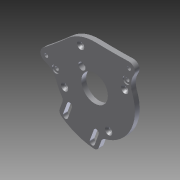
# Autodesk Inventor part: motor plate
Saved by Autodesk Inventor 2012 (Build 160160000, 160)
## iProperties
Created: 2012-02-08
Part Number: motor plate
Material: Default
Document SubType Name: Modeling
Designer: Antonella Wilby
Density: 1 g/cm^3
Author: Antonella Wilby
Autodesk Inventor part; units mm, degrees
ref_plane "YZ Plane" through (0, 0, 0) normal (1, 0, 0) x (0, 1, 0)
ref_plane "XZ Plane" through (0, 0, 0) normal (0, 1, 0) x (-1, 0, 0)
ref_plane "XY Plane" through (0, 0, 0) normal (0, 0, 1) x (1, 0, 0)
sketch "Sketch1" plane through (0, 0, 0) normal (0, 0, 1) x (1, 0, 0)
  line L0 (-661.6722, 0) -> (196.8414, 0) projected
  line L1 (0, -250.3433) -> (0, 987.2762) projected
  line L2 (0, 0) -> (-137.5064, 137.5064) construction
  circle A0 centre (0, 0) radius 17.78
  line L3 (0, 0) -> (46.0238, 46.0238) construction
  line L4 (-64.8398, 5.6727) -> (0, 0) construction
  circle A1 centre (-64.8398, 5.6727) radius 6.35 construction
  circle A2 centre (46.0238, 46.0238) radius 6.35 construction
  arc A3 (52.7316, 41.7801) -> (45.7909, 53.9579) centre (46.0238, 46.0238) ccw
  arc A4 (-69.7613, 11.9003) -> (-67.2505, -1.8898) centre (-64.8398, 5.6727) ccw
  line L5 (0, 0) -> (3.2586, 111.9917) construction
  line L6 (0, 0) -> (-89.6909, 100.7848) construction
  arc A5 (-69.7613, 11.9003) -> (-35.8824, 40.3207) centre (-539.0274, 605.7002) ccw
  arc A6 (1.5698, 53.9522) -> (45.7909, 53.9579) centre (23.5824, 810.4734) ccw
  arc A7 (-50.976, -17.7412) -> (-67.2505, -1.8898) centre (-74.9647, -26.0901) ccw
  arc A8 (52.7316, 41.7801) -> (50.4537, 19.1761) centre (74.1966, 28.2002) ccw
  arc A9 (1.5698, 53.9522) -> (-35.8824, 40.3207) centre (0, 0) ccw
  line L7 (-43.1182, -37.2395) -> (-46.8396, -47.4638)
  line L8 (9.0934, -56.243) -> (5.3721, -66.4673)
  arc A10 (-44.5419, -54.8181) -> (-1.1153, -70.6241) centre (6.0603, 16.6506) ccw
  arc A11 (-50.976, -17.7412) -> (-43.9184, -31.3763) centre (0, 0) ccw
  arc A12 (13.4752, -52.2659) -> (50.4537, 19.1761) centre (0, 0) ccw
  line L9 (-23.8901, -65.6375) -> (0, 0) construction
  arc A13 (-43.1182, -37.2395) -> (-43.9184, -31.3763) centre (-49.0853, -35.0676) ccw
  arc A14 (13.4752, -52.2659) -> (9.0934, -56.243) centre (15.0605, -58.4148) ccw
  arc A15 (-1.1153, -70.6241) -> (5.3721, -66.4673) centre (-0.595, -64.2955) ccw
  arc A16 (-46.8396, -47.4638) -> (-44.5419, -54.8181) centre (-40.8726, -49.6356) ccw
  circle A17 centre (-17.0625, 17.0625) radius 4.7625
  circle A18 centre (0, 0) radius 16.51 construction
  point P0 (-41.9333, -33.9838)
  point P1 (-48.4488, -51.885)
  point P2 (3.7629, -70.8885)
  point P3 (10.2784, -52.9873)
  dimension "d1" = 45
  dimension "d2" = 35.56
  dimension "d33" = 45
  dimension "d34" = 65.0875
  dimension "d39" = 65.0875
  dimension "d40" = 12.7
  dimension "d41" = 130
  dimension "d42" = 1.5875
  dimension "d43" = 1.5875
  dimension "d44" = 43.333
  dimension "d46" = 86.667
  dimension "d47" = 25.4
  dimension "d48" = 53.975
  dimension "d70" = 53.975
  dimension "d71" = 53.975
  dimension "d72" = 20
  dimension "d74" = 19.05
  dimension "d75" = 19.05
  dimension "d76" = 69.85
  dimension "d77" = 27.7812
  dimension "d78" = 6.35
  dimension "d89" = 24.13
  dimension "d90" = 9.525
  dimension "d91" = 33.02
  constraints: 35 point on circle, 19 centre point, 16 end point, 15 tangent, 7 point on line, 6 equal radius, 5 coincident, 2 parallel
  measures "d1" angle of L1 L2
  measures "d2" diameter of A0
  measures "d33" angle of L0 L3
  measures "d34" distance of L3.start L3.end
  measures "d39" distance of L4.start L3.start
  measures "d40" diameter of A1
  measures "d41" angle of L3 L4
  measures "d42" radial gap between concentric circles of A4 A1
  measures "d43" radial gap between concentric circles of A3 A2
  measures "d44" angle of L5 L3
  measures "d46" angle of L6 L3
  measures "d47" radius of A7
  measures "d48" radius of A9
  measures "d70" radius of A11
  measures "d71" radius of A12
  measures "d72" angle of L1 L8
  measures "d74" distance of point (-41.933, -33.984) point (-48.449, -51.885)
  measures "d75" distance of point (10.278, -52.987) point (3.763, -70.888)
  measures "d76" distance of L9.start L3.start
  measures "d77" distance between parallel lines of L9 L8
  measures "d78" radius of A13
  measures "d89" distance of point (0, 0) A17.centre
  measures "d90" diameter of A17
  measures "d91" diameter of A18
extrude "Base" add sketch "Sketch1" along normal mid plane 6.35 contours A4 A5 A9 L1 A0 L0 | L0 A0 L1 A15 A10 A16 L7 A13 A11 A7 A4 | L1 A9 A6 A3 A8 A12 L0 A0 | A0 L0 A12 A14 L8 A15 L1
sketch "Sketch3" plane through (0, 0, 3.175) normal (0, 0, 1) x (1, 0, 0)
  line L0 (0, 0) -> (-18.7854, 40.2854) construction
  line L1 (-98.1278, 0) -> (79.3255, 0) projected
  line L2 (0, -95.5696) -> (0, 78.8991) projected
  point P0 (-40.2854, -18.7854)
  point P1 (18.7854, -40.2854)
  point P2 (40.2854, 18.7854)
  dimension "d20" = 44.45
  dimension "d23" = 360
  dimension "d57" = 25
  constraints: 2 end point, 1 coincident, 5 other
  measures "d20" distance of L0.start L0.end
  measures "d57" angle of L2 L0
hole "Motor Mount Holes" at (-18.7854, 40.2854, 3.175) at (-40.2854, -18.7854, 3.175) at (18.7854, -40.2854, 3.175) at (40.2854, 18.7854, 3.175) direction (0, 0, -1) diameter 5.1054 end through all countersink diameter 9.779 countersink angle 82 clearance for "Flat Head Machine Screw (82)" size "#10" standard "Ansi Unified Screw Threads"
sketch "Sketch4" plane through (0, 0, -3.175) normal (0, 0, -1) x (-1, 0, 0)
  arc A0 (67.2505, -1.8898) -> (69.7613, 11.9003) centre (64.8398, 5.6727) ccw projected
  arc A1 (-45.7909, 53.9579) -> (-52.7316, 41.7801) centre (-46.0238, 46.0238) ccw projected
  constraints: 2 coincident
hole "Standoff holes to back plate" at (46.0238, 46.0238, -3.175) at (-64.8398, 5.6727, -3.175) direction (0, 0, 1) diameter 5.1054 end through all counterbore diameter 9.779 counterbore depth 1.5875 clearance for "Flat Head Machine Screw (82)" size "#10" standard "Ansi Unified Screw Threads"
sketch "Sketch5" plane through (0, 0, 3.175) normal (0, 0, 1) x (1, 0, 0)
  circle A0 centre (-64.8398, 5.6727) radius 2.5527 projected
  circle A1 centre (46.0238, 46.0238) radius 2.5527 projected
  arc A2 (-50.976, -17.7412) -> (-67.2505, -1.8898) centre (-74.9647, -26.0901) ccw projected
  arc A3 (52.7316, 41.7801) -> (50.4537, 19.1761) centre (74.1966, 28.2002) ccw projected
  circle A4 centre (-52.2111, -3.9465) radius 6.35 construction
  circle A5 centre (42.5328, 30.5374) radius 6.35 construction
  dimension "d58" = 15.875
  dimension "d59" = 15.875
  dimension "d60" = 12.7
  dimension "d62" = 12.7
  constraints: 2 centre point, 2 coincident, 2 tangent
  measures "d58" distance of A0.centre point (-52.211, -3.947)
  measures "d59" distance of point (42.533, 30.537) A1.centre
  measures "d60" diameter of A4
  measures "d62" diameter of A5
hole "Standoff holes to front plate" at (-52.2111, -3.9465, 3.175) at (42.5328, 30.5374, 3.175) direction (0, 0, -1) diameter 5.1054 end through all counterbore diameter 9.779 counterbore depth 1.5875 clearance for "Flat Head Machine Screw (82)" size "#10" standard "Ansi Unified Screw Threads"
sketch "Sketch6" plane through (0, 0, 3.175) normal (0, 0, 1) x (1, 0, 0)
  arc A0 (-44.5419, -54.8181) -> (-1.1153, -70.6241) centre (6.0603, 16.6506) ccw projected
  line L0 (9.0934, -56.243) -> (5.3721, -66.4673) projected
  arc A1 (-42.2267, -50.4413) -> (-35.8778, -52.7521) centre (-39.0522, -51.5967) ccw
  arc A2 (-6.4244, -63.4722) -> (-0.0755, -65.7831) centre (-3.25, -64.6276) ccw
  arc A3 (5.3541, -50.8654) -> (-0.9949, -48.5546) centre (2.1796, -49.71) ccw
  line L1 (-42.2267, -50.4413) -> (-36.7971, -35.5236)
  line L2 (-30.4482, -37.8345) -> (-35.8778, -52.7521)
  line L3 (-6.4244, -63.4722) -> (-0.9949, -48.5546)
  line L4 (5.3541, -50.8654) -> (-0.0755, -65.7831)
  line L5 (-39.0522, -51.5967) -> (-3.25, -64.6276) construction
  arc A4 (-30.4482, -37.8345) -> (-36.7971, -35.5236) centre (-33.6227, -36.6791) ccw
  dimension "d80" = 15.875
  dimension "d81" = 6.7564
  dimension "d82" = 5.353
  dimension "d83" = 38.1
  dimension "d84" = 2.3813
  dimension "d86" = 15.875
  constraints: 10 end point, 8 point on circle, 8 tangent, 4 centre point, 3 parallel, 2 point on line, 1 equal radius, 1 perpendicular
  measures "d80" distance of L3.start L3.end
  measures "d81" distance between parallel lines of L3 L4
  measures "d82" distance between parallel lines of L4 L0
  measures "d83" distance of L5.start L5.end
  measures "d86" distance of L1.start L1.end
extrude "Tensioning Slots" cut sketch "Sketch6" against normal through all
equation "\"d43\" = d42"
equation "\"d44\" = 0.333333 * d41"
equation "\"d46\" = 0.666667 * d41"
equation "\"d59\" = d58"
body "Solid1"
